Autodesk Inventor part; units mm, degrees
(part 3 of 4)
  spline S572 degree 2 poles (48.1472, 10.9048) (48.1472, 10.1779) (47.354, 9.3436) (46.6302, 9.3436) knots 0 0 0 1 2 2 2
  spline S573 degree 2 poles (46.6302, 9.3436) (45.9096, 9.3436) (45.11, 10.1779) (45.11, 10.9048) knots 0 0 0 1 2 2 2
  spline S574 degree 2 poles (45.11, 10.9048) (45.11, 11.6381) (45.9096, 12.4693) (46.6302, 12.4693) knots 0 0 0 1 2 2 2
  spline S575 degree 2 poles (46.6302, 12.4693) (47.3508, 12.4693) (48.1472, 11.6349) (48.1472, 10.9048) knots 0 0 0 1 2 2 2
  spline S576 degree 2 poles (47.2086, 10.8985) (47.2086, 11.1608) (47.1233, 11.5116) (47.0474, 11.6159) knots 0 0 0 1 2 2 2
  spline S577 degree 2 poles (47.0474, 11.6159) (46.9652, 11.7265) (46.7598, 11.8119) (46.6302, 11.8119) knots 0 0 0 1 2 2 2
  spline S578 degree 2 poles (46.6302, 11.8119) (46.5038, 11.8119) (46.3047, 11.736) (46.2225, 11.6286) knots 0 0 0 1 2 2 2
  spline S579 degree 2 poles (46.2225, 11.6286) (46.1435, 11.5274) (46.0487, 11.1703) (46.0487, 10.8985) knots 0 0 0 1 2 2 2
  spline S580 degree 2 poles (46.0487, 10.8985) (46.0487, 10.6299) (46.1372, 10.298) (46.2099, 10.1969) knots 0 0 0 1 2 2 2
  spline S581 degree 2 poles (46.2099, 10.1969) (46.2826, 10.0958) (46.5038, 10.0009) (46.6365, 10.0009) knots 0 0 0 1 2 2 2
  spline S582 degree 2 poles (46.6365, 10.0009) (46.7472, 10.0009) (46.9747, 10.0958) (47.0442, 10.1906) knots 0 0 0 1 2 2 2
  spline S583 degree 2 poles (47.0442, 10.1906) (47.1233, 10.3012) (47.2086, 10.6204) (47.2086, 10.8985) knots 0 0 0 1 2 2 2
  spline S584 degree 2 poles (53.3746, 10.6299) (53.3746, 10.3391) (53.1534, 9.8998) (52.9701, 9.7544) knots 0 0 0 1 2 2 2
  spline S585 degree 2 poles (52.9701, 9.7544) (52.7489, 9.5806) (52.2242, 9.4352) (51.8165, 9.4352) knots 0 0 0 1 2 2 2
  line L517 (51.8165, 9.4352) -> (50.2584, 9.4352)
  line L518 (50.2584, 9.4352) -> (50.2584, 13.3352)
  line L519 (50.2584, 13.3352) -> (51.6332, 13.3352)
  spline S586 degree 2 poles (51.6332, 13.3352) (52.063, 13.3352) (52.5055, 13.2689) (52.6983, 13.1646) knots 0 0 0 1 2 2 2
  spline S587 degree 2 poles (52.6983, 13.1646) (52.91, 13.0539) (53.1155, 12.6747) (53.1155, 12.4282) knots 0 0 0 1 2 2 2
  spline S588 degree 2 poles (53.1155, 12.4282) (53.1155, 12.1437) (52.831, 11.6981) (52.5782, 11.5938) knots 0 0 0 1 2 2 2
  line L520 (52.5782, 11.5938) -> (52.5782, 11.5748)
  spline S589 degree 2 poles (52.5782, 11.5748) (52.9417, 11.499) (53.3746, 11.0281) (53.3746, 10.6299) knots 0 0 0 1 2 2 2
  spline S590 degree 2 poles (52.3633, 10.6457) (52.3633, 10.829) (52.2179, 11.0344) (52.0725, 11.0881) knots 0 0 0 1 2 2 2
  spline S591 degree 2 poles (52.0725, 11.0881) (51.984, 11.1229) (51.6711, 11.1292) (51.412, 11.1292) knots 0 0 0 1 2 2 2
  line L521 (51.412, 11.1292) -> (51.2318, 11.1292)
  line L522 (51.2318, 11.1292) -> (51.2318, 10.1463)
  line L523 (51.2318, 10.1463) -> (51.2856, 10.1463)
  spline S592 degree 2 poles (51.2856, 10.1463) (51.6648, 10.1463) (51.9556, 10.1558) (52.1073, 10.2222) knots 0 0 0 1 2 2 2
  spline S593 degree 2 poles (52.1073, 10.2222) (52.24, 10.2822) (52.3633, 10.5035) (52.3633, 10.6457) knots 0 0 0 1 2 2 2
  spline S594 degree 2 poles (52.1199, 12.2354) (52.1199, 12.3302) (52.022, 12.5293) (51.9208, 12.5736) knots 0 0 0 1 2 2 2
  spline S595 degree 2 poles (51.9208, 12.5736) (51.826, 12.6178) (51.5605, 12.6241) (51.2982, 12.6241) knots 0 0 0 1 2 2 2
  line L524 (51.2982, 12.6241) -> (51.2318, 12.6241)
  line L525 (51.2318, 12.6241) -> (51.2318, 11.7961)
  line L526 (51.2318, 11.7961) -> (51.3551, 11.7961)
  spline S596 degree 2 poles (51.3551, 11.7961) (51.6048, 11.7961) (51.807, 11.8056) (51.9145, 11.8561) knots 0 0 0 1 2 2 2
  spline S597 degree 2 poles (51.9145, 11.8561) (52.0314, 11.913) (52.1199, 12.1058) (52.1199, 12.2354) knots 0 0 0 1 2 2 2
  spline S598 degree 2 poles (55.391, 9.3562) (54.5566, 9.3562) (53.6686, 10.1526) (53.6686, 10.889) knots 0 0 0 1 2 2 2
  spline S599 degree 2 poles (53.6686, 10.889) (53.6686, 11.6096) (54.4966, 12.4693) (55.2425, 12.4693) knots 0 0 0 1 2 2 2
  spline S600 degree 2 poles (55.2425, 12.4693) (55.9156, 12.4693) (56.5983, 11.7392) (56.5983, 11.0629) knots 0 0 0 1 2 2 2
  line L527 (56.5983, 11.0629) -> (56.5983, 10.731)
  line L528 (56.5983, 10.731) -> (54.5851, 10.731)
  spline S601 degree 2 poles (54.5851, 10.731) (54.5977, 10.5256) (54.7463, 10.2538) (54.8664, 10.1716) knots 0 0 0 1 2 2 2
  spline S602 degree 2 poles (54.8664, 10.1716) (54.9833, 10.0894) (55.2994, 10.0199) (55.4858, 10.0199) knots 0 0 0 1 2 2 2
  spline S603 degree 2 poles (55.4858, 10.0199) (55.6438, 10.0199) (55.9536, 10.0894) (56.0831, 10.1495) knots 0 0 0 1 2 2 2
  spline S604 degree 2 poles (56.0831, 10.1495) (56.1969, 10.1969) (56.3865, 10.3138) (56.4466, 10.3581) knots 0 0 0 1 2 2 2
  line L529 (56.4466, 10.3581) -> (56.5446, 10.3581)
  line L530 (56.5446, 10.3581) -> (56.5446, 9.5996)
  spline S605 degree 2 poles (56.5446, 9.5996) (56.4308, 9.5553) (56.2475, 9.4795) (56.0831, 9.4415) knots 0 0 0 1 2 2 2
  spline S606 degree 2 poles (56.0831, 9.4415) (55.9346, 9.4005) (55.6186, 9.3562) (55.391, 9.3562) knots 0 0 0 1 2 2 2
  spline S607 degree 2 poles (55.6944, 11.2841) (55.6881, 11.5748) (55.4321, 11.8814) (55.1698, 11.8814) knots 0 0 0 1 2 2 2
  spline S608 degree 2 poles (55.1698, 11.8814) (54.9011, 11.8814) (54.5977, 11.559) (54.5819, 11.2841) knots 0 0 0 1 2 2 2
  line L531 (54.5819, 11.2841) -> (55.6944, 11.2841)
  line L532 (59.822, 9.4352) -> (58.8991, 9.4352)
  line L533 (58.8991, 9.4352) -> (58.8991, 10.8922)
  spline S609 degree 2 poles (58.8991, 10.8922) (58.8991, 11.0723) (58.8707, 11.4263) (58.8327, 11.5085) knots 0 0 0 1 2 2 2
  spline S610 degree 2 poles (58.8327, 11.5085) (58.7853, 11.6096) (58.6083, 11.6949) (58.4566, 11.6949) knots 0 0 0 1 2 2 2
  spline S611 degree 2 poles (58.4566, 11.6949) (58.346, 11.6949) (58.1153, 11.6096) (57.9857, 11.518) knots 0 0 0 1 2 2 2
  line L534 (57.9857, 11.518) -> (57.9857, 9.4352)
  line L535 (57.9857, 9.4352) -> (57.0692, 9.4352)
  line L536 (57.0692, 9.4352) -> (57.0692, 12.3776)
  line L537 (57.0692, 12.3776) -> (57.9857, 12.3776)
  line L538 (57.9857, 12.3776) -> (57.9857, 12.0521)
  spline S612 degree 2 poles (57.9857, 12.0521) (58.2101, 12.2417) (58.6368, 12.4566) (58.8959, 12.4566) knots 0 0 0 1 2 2 2
  spline S613 degree 2 poles (58.8959, 12.4566) (59.3447, 12.4566) (59.822, 11.8877) (59.822, 11.3505) knots 0 0 0 1 2 2 2
  line L539 (59.822, 11.3505) -> (59.822, 9.4352)
  spline S614 degree 2 poles (62.009, 9.3562) (61.1746, 9.3562) (60.2865, 10.1526) (60.2865, 10.889) knots 0 0 0 1 2 2 2
  spline S615 degree 2 poles (60.2865, 10.889) (60.2865, 11.6096) (61.1146, 12.4693) (61.8605, 12.4693) knots 0 0 0 1 2 2 2
  spline S616 degree 2 poles (61.8605, 12.4693) (62.5336, 12.4693) (63.2163, 11.7392) (63.2163, 11.0629) knots 0 0 0 1 2 2 2
  line L540 (63.2163, 11.0629) -> (63.2163, 10.731)
  line L541 (63.2163, 10.731) -> (61.2031, 10.731)
  spline S617 degree 2 poles (61.2031, 10.731) (61.2157, 10.5256) (61.3643, 10.2538) (61.4844, 10.1716) knots 0 0 0 1 2 2 2
  spline S618 degree 2 poles (61.4844, 10.1716) (61.6013, 10.0894) (61.9173, 10.0199) (62.1038, 10.0199) knots 0 0 0 1 2 2 2
  spline S619 degree 2 poles (62.1038, 10.0199) (62.2618, 10.0199) (62.5716, 10.0894) (62.7011, 10.1495) knots 0 0 0 1 2 2 2
  spline S620 degree 2 poles (62.7011, 10.1495) (62.8149, 10.1969) (63.0045, 10.3138) (63.0646, 10.3581) knots 0 0 0 1 2 2 2
  line L542 (63.0646, 10.3581) -> (63.1626, 10.3581)
  line L543 (63.1626, 10.3581) -> (63.1626, 9.5996)
  spline S621 degree 2 poles (63.1626, 9.5996) (63.0488, 9.5553) (62.8655, 9.4795) (62.7011, 9.4415) knots 0 0 0 1 2 2 2
  spline S622 degree 2 poles (62.7011, 9.4415) (62.5526, 9.4005) (62.2365, 9.3562) (62.009, 9.3562) knots 0 0 0 1 2 2 2
  spline S623 degree 2 poles (62.3124, 11.2841) (62.3061, 11.5748) (62.0501, 11.8814) (61.7878, 11.8814) knots 0 0 0 1 2 2 2
  spline S624 degree 2 poles (61.7878, 11.8814) (61.5191, 11.8814) (61.2157, 11.559) (61.1999, 11.2841) knots 0 0 0 1 2 2 2
  line L544 (61.1999, 11.2841) -> (62.3124, 11.2841)
  line L545 (66.3609, 9.4352) -> (65.4444, 9.4352)
  line L546 (65.4444, 9.4352) -> (65.4444, 9.7418)
  spline S625 degree 2 poles (65.4444, 9.7418) (65.3559, 9.6691) (65.1284, 9.5016) (65.0399, 9.4573) knots 0 0 0 1 2 2 2
  spline S626 degree 2 poles (65.0399, 9.4573) (64.9324, 9.4068) (64.7175, 9.353) (64.569, 9.353) knots 0 0 0 1 2 2 2
  spline S627 degree 2 poles (64.569, 9.353) (64.0664, 9.353) (63.4786, 10.1874) (63.4786, 10.8827) knots 0 0 0 1 2 2 2
  spline S628 degree 2 poles (63.4786, 10.8827) (63.4786, 11.2683) (63.6777, 11.834) (63.8515, 12.0426) knots 0 0 0 1 2 2 2
  spline S629 degree 2 poles (63.8515, 12.0426) (64.0127, 12.2354) (64.4678, 12.4566) (64.7207, 12.4566) knots 0 0 0 1 2 2 2
  spline S630 degree 2 poles (64.7207, 12.4566) (64.9514, 12.4566) (65.2485, 12.3586) (65.4444, 12.2575) knots 0 0 0 1 2 2 2
  line L547 (65.4444, 12.2575) -> (65.4444, 13.509)
  line L548 (65.4444, 13.509) -> (66.3609, 13.509)
  line L549 (66.3609, 13.509) -> (66.3609, 9.4352)
  line L550 (65.4444, 10.2443) -> (65.4444, 11.6886)
  spline S631 degree 2 poles (65.4444, 11.6886) (65.378, 11.7234) (65.1568, 11.7676) (65.0778, 11.7676) knots 0 0 0 1 2 2 2
  spline S632 degree 2 poles (65.0778, 11.7676) (64.7491, 11.7676) (64.4173, 11.3062) (64.4173, 10.8922) knots 0 0 0 1 2 2 2
  spline S633 degree 2 poles (64.4173, 10.8922) (64.4173, 10.456) (64.6827, 10.0673) (64.9767, 10.0673) knots 0 0 0 1 2 2 2
  spline S634 degree 2 poles (64.9767, 10.0673) (65.0968, 10.0673) (65.3433, 10.1621) (65.4444, 10.2443) knots 0 0 0 1 2 2 2
  line L551 (69.7932, 9.4352) -> (68.8767, 9.4352)
  line L552 (68.8767, 9.4352) -> (68.8767, 9.7607)
  spline S635 degree 2 poles (68.8767, 9.7607) (68.6396, 9.5616) (68.2414, 9.353) (67.9664, 9.353) knots 0 0 0 1 2 2 2
  spline S636 degree 2 poles (67.9664, 9.353) (67.5303, 9.353) (67.0404, 9.9061) (67.0404, 10.4624) knots 0 0 0 1 2 2 2
  line L553 (67.0404, 10.4624) -> (67.0404, 12.3776)
  line L554 (67.0404, 12.3776) -> (67.9633, 12.3776)
  line L555 (67.9633, 12.3776) -> (67.9633, 10.9175)
  spline S637 degree 2 poles (67.9633, 10.9175) (67.9633, 10.6899) (67.9854, 10.3992) (68.0297, 10.3012) knots 0 0 0 1 2 2 2
  spline S638 degree 2 poles (68.0297, 10.3012) (68.0739, 10.2095) (68.2477, 10.1147) (68.4058, 10.1147) knots 0 0 0 1 2 2 2
  spline S639 degree 2 poles (68.4058, 10.1147) (68.5006, 10.1147) (68.766, 10.2095) (68.8767, 10.2917) knots 0 0 0 1 2 2 2
  line L556 (68.8767, 10.2917) -> (68.8767, 12.3776)
  line L557 (68.8767, 12.3776) -> (69.7932, 12.3776)
  line L558 (69.7932, 12.3776) -> (69.7932, 9.4352)
  spline S640 degree 2 poles (71.936, 9.3562) (71.5725, 9.3562) (70.9689, 9.5395) (70.7445, 9.7291) knots 0 0 0 1 2 2 2
  spline S641 degree 2 poles (70.7445, 9.7291) (70.5264, 9.9219) (70.2799, 10.5003) (70.2799, 10.8922) knots 0 0 0 1 2 2 2
  spline S642 degree 2 poles (70.2799, 10.8922) (70.2799, 11.3157) (70.5454, 11.9067) (70.7761, 12.0963) knots 0 0 0 1 2 2 2
  spline S643 degree 2 poles (70.7761, 12.0963) (70.9942, 12.2796) (71.5883, 12.4566) (71.9107, 12.4566) knots 0 0 0 1 2 2 2
  spline S644 degree 2 poles (71.9107, 12.4566) (72.1541, 12.4566) (72.6408, 12.3428) (72.8873, 12.2196) knots 0 0 0 1 2 2 2
  line L559 (72.8873, 12.2196) -> (72.8873, 11.4358)
  line L560 (72.8873, 11.4358) -> (72.7703, 11.4358)
  spline S645 degree 2 poles (72.7703, 11.4358) (72.7135, 11.4895) (72.5554, 11.6159) (72.4606, 11.6665) knots 0 0 0 1 2 2 2
  spline S646 degree 2 poles (72.4606, 11.6665) (72.3595, 11.7234) (72.1098, 11.7992) (71.9549, 11.7992) knots 0 0 0 1 2 2 2
  spline S647 degree 2 poles (71.9549, 11.7992) (71.6041, 11.7992) (71.2186, 11.3094) (71.2186, 10.8922) knots 0 0 0 1 2 2 2
  spline S648 degree 2 poles (71.2186, 10.8922) (71.2186, 10.4497) (71.6294, 10.0136) (71.9707, 10.0136) knots 0 0 0 1 2 2 2
  spline S649 degree 2 poles (71.9707, 10.0136) (72.1446, 10.0136) (72.4037, 10.0926) (72.4985, 10.1495) knots 0 0 0 1 2 2 2
  spline S650 degree 2 poles (72.4985, 10.1495) (72.5902, 10.2032) (72.7229, 10.3233) (72.7703, 10.3707) knots 0 0 0 1 2 2 2
  line L561 (72.7703, 10.3707) -> (72.8873, 10.3707)
  line L562 (72.8873, 10.3707) -> (72.8873, 9.5838)
  spline S651 degree 2 poles (72.8873, 9.5838) (72.8083, 9.549) (72.6028, 9.4605) (72.4954, 9.4321) knots 0 0 0 1 2 2 2
  spline S652 degree 2 poles (72.4954, 9.4321) (72.3626, 9.3941) (72.1288, 9.3562) (71.936, 9.3562) knots 0 0 0 1 2 2 2
  spline S653 degree 2 poles (74.831, 9.3562) (73.9966, 9.3562) (73.1085, 10.1526) (73.1085, 10.889) knots 0 0 0 1 2 2 2
  spline S654 degree 2 poles (73.1085, 10.889) (73.1085, 11.6096) (73.9365, 12.4693) (74.6824, 12.4693) knots 0 0 0 1 2 2 2
  spline S655 degree 2 poles (74.6824, 12.4693) (75.3556, 12.4693) (76.0382, 11.7392) (76.0382, 11.0629) knots 0 0 0 1 2 2 2
  line L563 (76.0382, 11.0629) -> (76.0382, 10.731)
  line L564 (76.0382, 10.731) -> (74.025, 10.731)
  spline S656 degree 2 poles (74.025, 10.731) (74.0377, 10.5256) (74.1862, 10.2538) (74.3063, 10.1716) knots 0 0 0 1 2 2 2
  spline S657 degree 2 poles (74.3063, 10.1716) (74.4233, 10.0894) (74.7393, 10.0199) (74.9258, 10.0199) knots 0 0 0 1 2 2 2
  spline S658 degree 2 poles (74.9258, 10.0199) (75.0838, 10.0199) (75.3935, 10.0894) (75.5231, 10.1495) knots 0 0 0 1 2 2 2
  spline S659 degree 2 poles (75.5231, 10.1495) (75.6369, 10.1969) (75.8265, 10.3138) (75.8865, 10.3581) knots 0 0 0 1 2 2 2
  line L565 (75.8865, 10.3581) -> (75.9845, 10.3581)
  line L566 (75.9845, 10.3581) -> (75.9845, 9.5996)
  spline S660 degree 2 poles (75.9845, 9.5996) (75.8707, 9.5553) (75.6874, 9.4795) (75.5231, 9.4415) knots 0 0 0 1 2 2 2
  spline S661 degree 2 poles (75.5231, 9.4415) (75.3746, 9.4005) (75.0585, 9.3562) (74.831, 9.3562) knots 0 0 0 1 2 2 2
  spline S662 degree 2 poles (75.1344, 11.2841) (75.128, 11.5748) (74.872, 11.8814) (74.6097, 11.8814) knots 0 0 0 1 2 2 2
  spline S663 degree 2 poles (74.6097, 11.8814) (74.3411, 11.8814) (74.0377, 11.559) (74.0219, 11.2841) knots 0 0 0 1 2 2 2
  line L567 (74.0219, 11.2841) -> (75.1344, 11.2841)
  line L568 (81.4742, 9.4352) -> (80.5324, 9.4352)
  line L569 (80.5324, 9.4352) -> (79.028, 12.1532)
  line L570 (79.028, 12.1532) -> (79.028, 9.4352)
  line L571 (79.028, 9.4352) -> (78.1336, 9.4352)
  line L572 (78.1336, 9.4352) -> (78.1336, 13.3352)
  line L573 (78.1336, 13.3352) -> (79.3346, 13.3352)
  line L574 (79.3346, 13.3352) -> (80.5798, 11.1008)
  line L575 (80.5798, 11.1008) -> (80.5798, 13.3352)
  line L576 (80.5798, 13.3352) -> (81.4742, 13.3352)
  line L577 (81.4742, 13.3352) -> (81.4742, 9.4352)
  spline S664 degree 2 poles (83.7213, 9.3562) (82.887, 9.3562) (81.9989, 10.1526) (81.9989, 10.889) knots 0 0 0 1 2 2 2
  spline S665 degree 2 poles (81.9989, 10.889) (81.9989, 11.6096) (82.8269, 12.4693) (83.5728, 12.4693) knots 0 0 0 1 2 2 2
  spline S666 degree 2 poles (83.5728, 12.4693) (84.2459, 12.4693) (84.9286, 11.7392) (84.9286, 11.0629) knots 0 0 0 1 2 2 2
  line L578 (84.9286, 11.0629) -> (84.9286, 10.731)
  line L579 (84.9286, 10.731) -> (82.9154, 10.731)
  spline S667 degree 2 poles (82.9154, 10.731) (82.928, 10.5256) (83.0766, 10.2538) (83.1967, 10.1716) knots 0 0 0 1 2 2 2
  spline S668 degree 2 poles (83.1967, 10.1716) (83.3136, 10.0894) (83.6297, 10.0199) (83.8161, 10.0199) knots 0 0 0 1 2 2 2
  spline S669 degree 2 poles (83.8161, 10.0199) (83.9741, 10.0199) (84.2839, 10.0894) (84.4135, 10.1495) knots 0 0 0 1 2 2 2
  spline S670 degree 2 poles (84.4135, 10.1495) (84.5272, 10.1969) (84.7169, 10.3138) (84.7769, 10.3581) knots 0 0 0 1 2 2 2
  line L580 (84.7769, 10.3581) -> (84.8749, 10.3581)
  line L581 (84.8749, 10.3581) -> (84.8749, 9.5996)
  spline S671 degree 2 poles (84.8749, 9.5996) (84.7611, 9.5553) (84.5778, 9.4795) (84.4135, 9.4415) knots 0 0 0 1 2 2 2
  spline S672 degree 2 poles (84.4135, 9.4415) (84.2649, 9.4005) (83.9489, 9.3562) (83.7213, 9.3562) knots 0 0 0 1 2 2 2
  spline S673 degree 2 poles (84.0247, 11.2841) (84.0184, 11.5748) (83.7624, 11.8814) (83.5001, 11.8814) knots 0 0 0 1 2 2 2
  spline S674 degree 2 poles (83.5001, 11.8814) (83.2314, 11.8814) (82.928, 11.559) (82.9122, 11.2841) knots 0 0 0 1 2 2 2
  line L582 (82.9122, 11.2841) -> (84.0247, 11.2841)
  spline S675 degree 2 poles (86.5246, 9.3783) (85.9652, 9.3783) (85.4532, 9.8398) (85.4532, 10.3644) knots 0 0 0 1 2 2 2
  line L583 (85.4532, 10.3644) -> (85.4532, 11.7392)
  line L584 (85.4532, 11.7392) -> (85.1024, 11.7392)
  line L585 (85.1024, 11.7392) -> (85.1024, 12.3776)
  line L586 (85.1024, 12.3776) -> (85.4532, 12.3776)
  line L587 (85.4532, 12.3776) -> (85.4532, 13.2183)
  line L588 (85.4532, 13.2183) -> (86.3698, 13.2183)
  line L589 (86.3698, 13.2183) -> (86.3698, 12.3776)
  line L590 (86.3698, 12.3776) -> (87.2547, 12.3776)
  line L591 (87.2547, 12.3776) -> (87.2547, 11.7392)
  line L592 (87.2547, 11.7392) -> (86.3698, 11.7392)
  line L593 (86.3698, 11.7392) -> (86.3698, 10.6931)
  spline S676 degree 2 poles (86.3698, 10.6931) (86.3698, 10.5382) (86.3761, 10.3075) (86.414, 10.2159) knots 0 0 0 1 2 2 2
  spline S677 degree 2 poles (86.414, 10.2159) (86.4519, 10.1242) (86.6384, 10.0167) (86.8154, 10.0167) knots 0 0 0 1 2 2 2
  spline S678 degree 2 poles (86.8154, 10.0167) (86.8912, 10.0167) (87.1283, 10.08) (87.1757, 10.1052) knots 0 0 0 1 2 2 2
  line L594 (87.1757, 10.1052) -> (87.2547, 10.1052)
  line L595 (87.2547, 10.1052) -> (87.2547, 9.4605)
  spline S679 degree 2 poles (87.2547, 9.4605) (87.1062, 9.4226) (86.7711, 9.3783) (86.5246, 9.3783) knots 0 0 0 1 2 2 2
  spline S680 degree 2 poles (90.4499, 10.9048) (90.4499, 10.1779) (89.6566, 9.3436) (88.9329, 9.3436) knots 0 0 0 1 2 2 2
  spline S681 degree 2 poles (88.9329, 9.3436) (88.2123, 9.3436) (87.4127, 10.1779) (87.4127, 10.9048) knots 0 0 0 1 2 2 2
  spline S682 degree 2 poles (87.4127, 10.9048) (87.4127, 11.6381) (88.2123, 12.4693) (88.9329, 12.4693) knots 0 0 0 1 2 2 2
  spline S683 degree 2 poles (88.9329, 12.4693) (89.6535, 12.4693) (90.4499, 11.6349) (90.4499, 10.9048) knots 0 0 0 1 2 2 2
  spline S684 degree 2 poles (89.5113, 10.8985) (89.5113, 11.1608) (89.4259, 11.5116) (89.3501, 11.6159) knots 0 0 0 1 2 2 2
  spline S685 degree 2 poles (89.3501, 11.6159) (89.2679, 11.7265) (89.0625, 11.8119) (88.9329, 11.8119) knots 0 0 0 1 2 2 2
  spline S686 degree 2 poles (88.9329, 11.8119) (88.8065, 11.8119) (88.6074, 11.736) (88.5252, 11.6286) knots 0 0 0 1 2 2 2
  spline S687 degree 2 poles (88.5252, 11.6286) (88.4462, 11.5274) (88.3514, 11.1703) (88.3514, 10.8985) knots 0 0 0 1 2 2 2
  spline S688 degree 2 poles (88.3514, 10.8985) (88.3514, 10.6299) (88.4399, 10.298) (88.5126, 10.1969) knots 0 0 0 1 2 2 2
  spline S689 degree 2 poles (88.5126, 10.1969) (88.5852, 10.0958) (88.8065, 10.0009) (88.9392, 10.0009) knots 0 0 0 1 2 2 2
  spline S690 degree 2 poles (88.9392, 10.0009) (89.0498, 10.0009) (89.2774, 10.0958) (89.3469, 10.1906) knots 0 0 0 1 2 2 2
  spline S691 degree 2 poles (89.3469, 10.1906) (89.4259, 10.3012) (89.5113, 10.6204) (89.5113, 10.8985) knots 0 0 0 1 2 2 2
  line L596 (44.4187, 2.6614) -> (41.5521, 2.6614)
  line L597 (41.5521, 2.6614) -> (41.5521, 3.2967)
  spline S692 degree 2 poles (41.5521, 3.2967) (41.9156, 3.5874) (42.4971, 4.0994) (42.7152, 4.3302) knots 0 0 0 1 2 2 2
  spline S693 degree 2 poles (42.7152, 4.3302) (43.0028, 4.6304) (43.2588, 5.0887) (43.2588, 5.3289) knots 0 0 0 1 2 2 2
  spline S694 degree 2 poles (43.2588, 5.3289) (43.2588, 5.6007) (42.9333, 5.8914) (42.6425, 5.8914) knots 0 0 0 1 2 2 2
  spline S695 degree 2 poles (42.6425, 5.8914) (42.4939, 5.8914) (42.2285, 5.8187) (42.0926, 5.7618) knots 0 0 0 1 2 2 2
  spline S696 degree 2 poles (42.0926, 5.7618) (41.9598, 5.7018) (41.7702, 5.5754) (41.7228, 5.5438) knots 0 0 0 1 2 2 2
  line L598 (41.7228, 5.5438) -> (41.6469, 5.5438)
  line L599 (41.6469, 5.5438) -> (41.6469, 6.3939)
  spline S697 degree 2 poles (41.6469, 6.3939) (41.8113, 6.4729) (42.5129, 6.6373) (42.8384, 6.6373) knots 0 0 0 1 2 2 2
  spline S698 degree 2 poles (42.8384, 6.6373) (43.5337, 6.6373) (44.248, 6.0178) (44.248, 5.4584) knots 0 0 0 1 2 2 2
  spline S699 degree 2 poles (44.248, 5.4584) (44.248, 5.1139) (43.9225, 4.4502) (43.5464, 4.071) knots 0 0 0 1 2 2 2
  spline S700 degree 2 poles (43.5464, 4.071) (43.3093, 3.8371) (42.8637, 3.4737) (42.7657, 3.3978) knots 0 0 0 1 2 2 2
  line L600 (42.7657, 3.3978) -> (44.4187, 3.3978)
  line L601 (44.4187, 3.3978) -> (44.4187, 2.6614)
  spline S701 degree 2 poles (47.7845, 4.6114) (47.7845, 4.1058) (47.6234, 3.3473) (47.4432, 3.0913) knots 0 0 0 1 2 2 2
  spline S702 degree 2 poles (47.4432, 3.0913) (47.2662, 2.8384) (46.6942, 2.5793) (46.2833, 2.5793) knots 0 0 0 1 2 2 2
  spline S703 degree 2 poles (46.2833, 2.5793) (45.8693, 2.5793) (45.3004, 2.8384) (45.1203, 3.0976) knots 0 0 0 1 2 2 2
  spline S704 degree 2 poles (45.1203, 3.0976) (44.9401, 3.3536) (44.779, 4.1058) (44.779, 4.6114) knots 0 0 0 1 2 2 2
  spline S705 degree 2 poles (44.779, 4.6114) (44.779, 5.1297) (44.9401, 5.863) (45.1234, 6.1284) knots 0 0 0 1 2 2 2
  spline S706 degree 2 poles (45.1234, 6.1284) (45.3068, 6.3876) (45.8851, 6.6404) (46.2833, 6.6404) knots 0 0 0 1 2 2 2
  spline S707 degree 2 poles (46.2833, 6.6404) (46.7037, 6.6404) (47.2662, 6.375) (47.4464, 6.1126) knots 0 0 0 1 2 2 2
  spline S708 degree 2 poles (47.4464, 6.1126) (47.6234, 5.8567) (47.7845, 5.1013) (47.7845, 4.6114) knots 0 0 0 1 2 2 2
  spline S709 degree 2 poles (46.8016, 4.6114) (46.8016, 5.3352) (46.5646, 5.9199) (46.2833, 5.9199) knots 0 0 0 1 2 2 2
  spline S710 degree 2 poles (46.2833, 5.9199) (46.0021, 5.9199) (45.7619, 5.3352) (45.7619, 4.6083) knots 0 0 0 1 2 2 2
  spline S711 degree 2 poles (45.7619, 4.6083) (45.7619, 3.894) (46.0021, 3.2998) (46.2833, 3.2998) knots 0 0 0 1 2 2 2
  spline S712 degree 2 poles (46.2833, 3.2998) (46.5615, 3.2998) (46.8016, 3.894) (46.8016, 4.6114) knots 0 0 0 1 2 2 2
  line L602 (51.2516, 2.6614) -> (48.385, 2.6614)
  line L603 (48.385, 2.6614) -> (48.385, 3.2967)
  spline S713 degree 2 poles (48.385, 3.2967) (48.7485, 3.5874) (49.33, 4.0994) (49.5481, 4.3302) knots 0 0 0 1 2 2 2
  spline S714 degree 2 poles (49.5481, 4.3302) (49.8357, 4.6304) (50.0917, 5.0887) (50.0917, 5.3289) knots 0 0 0 1 2 2 2
  spline S715 degree 2 poles (50.0917, 5.3289) (50.0917, 5.6007) (49.7662, 5.8914) (49.4754, 5.8914) knots 0 0 0 1 2 2 2
  spline S716 degree 2 poles (49.4754, 5.8914) (49.3268, 5.8914) (49.0614, 5.8187) (48.9255, 5.7618) knots 0 0 0 1 2 2 2
  spline S717 degree 2 poles (48.9255, 5.7618) (48.7927, 5.7018) (48.6031, 5.5754) (48.5557, 5.5438) knots 0 0 0 1 2 2 2
  line L604 (48.5557, 5.5438) -> (48.4798, 5.5438)
  line L605 (48.4798, 5.5438) -> (48.4798, 6.3939)
  spline S718 degree 2 poles (48.4798, 6.3939) (48.6442, 6.4729) (49.3458, 6.6373) (49.6713, 6.6373) knots 0 0 0 1 2 2 2
  spline S719 degree 2 poles (49.6713, 6.6373) (50.3666, 6.6373) (51.0809, 6.0178) (51.0809, 5.4584) knots 0 0 0 1 2 2 2
  spline S720 degree 2 poles (51.0809, 5.4584) (51.0809, 5.1139) (50.7554, 4.4502) (50.3793, 4.071) knots 0 0 0 1 2 2 2
  spline S721 degree 2 poles (50.3793, 4.071) (50.1422, 3.8371) (49.6966, 3.4737) (49.5986, 3.3978) knots 0 0 0 1 2 2 2
  line L606 (49.5986, 3.3978) -> (51.2516, 3.3978)
  line L607 (51.2516, 3.3978) -> (51.2516, 2.6614)
  line L608 (54.668, 2.6614) -> (51.8015, 2.6614)
  line L609 (51.8015, 2.6614) -> (51.8015, 3.2967)
  spline S722 degree 2 poles (51.8015, 3.2967) (52.1649, 3.5874) (52.7465, 4.0994) (52.9645, 4.3302) knots 0 0 0 1 2 2 2
  spline S723 degree 2 poles (52.9645, 4.3302) (53.2521, 4.6304) (53.5081, 5.0887) (53.5081, 5.3289) knots 0 0 0 1 2 2 2
  spline S724 degree 2 poles (53.5081, 5.3289) (53.5081, 5.6007) (53.1826, 5.8914) (52.8918, 5.8914) knots 0 0 0 1 2 2 2
  spline S725 degree 2 poles (52.8918, 5.8914) (52.7433, 5.8914) (52.4778, 5.8187) (52.3419, 5.7618) knots 0 0 0 1 2 2 2
  spline S726 degree 2 poles (52.3419, 5.7618) (52.2092, 5.7018) (52.0196, 5.5754) (51.9721, 5.5438) knots 0 0 0 1 2 2 2
  line L610 (51.9721, 5.5438) -> (51.8963, 5.5438)
  line L611 (51.8963, 5.5438) -> (51.8963, 6.3939)
  spline S727 degree 2 poles (51.8963, 6.3939) (52.0606, 6.4729) (52.7623, 6.6373) (53.0878, 6.6373) knots 0 0 0 1 2 2 2
  spline S728 degree 2 poles (53.0878, 6.6373) (53.7831, 6.6373) (54.4974, 6.0178) (54.4974, 5.4584) knots 0 0 0 1 2 2 2
  spline S729 degree 2 poles (54.4974, 5.4584) (54.4974, 5.1139) (54.1718, 4.4502) (53.7957, 4.071) knots 0 0 0 1 2 2 2
  spline S730 degree 2 poles (53.7957, 4.071) (53.5587, 3.8371) (53.1131, 3.4737) (53.0151, 3.3978) knots 0 0 0 1 2 2 2
  line L612 (53.0151, 3.3978) -> (54.668, 3.3978)
  line L613 (54.668, 3.3978) -> (54.668, 2.6614)
  point P0 (0, 0)
  constraints: 10 other
extrude "Extrusão3" cut sketch "Esboço2" against normal blind 0.8
chamfer "Chanfro1" distance 4 angle 45 4 edges at (1, 40, -100) (1, 0, -100) (1, 40, 0) (1, 0, 0)
fillet "Arredondamento1" radius 2 8 edges at (1, 40, -4) (1, 36, 0) (1, 4, 0) (1, 0, -4) (1, 0, -96) (1, 4, -100) (1, 36, -100) (1, 40, -96)
sketch "Esboço4" plane through (2, 0, 0) normal (1, 0, 0) x (0, 0, -1)
  line L0 (45.497, 3.0913) -> (45.497, 2.5793) projected
  line L1 (46.2833, 8.4074) -> (45.1203, 8.4074) projected
  line L2 (45.0667, 6.1126) -> (45.0667, 4.6114) projected
  line L3 (47.7845, 11.4269) -> (47.4432, 11.4269) projected
  line L4 (88.9329, 10.6586) -> (88.5252, 10.6586) projected
  line L5 (50.5558, 25.9389) -> (50.2933, 25.2422) projected
  line L6 (88.3514, 8.4074) -> (88.5126, 8.4074) projected
  line L7 (49.6589, 25.5886) -> (49.6742, 25.6323) projected
  line L8 (40.3066, 9.4415) -> (40.3066, 9.3562) projected
  line L9 (83.7213, 8.4074) -> (81.9989, 8.4074) projected
  line L10 (84.8749, 10.3581) -> (84.8749, 9.5996) projected
  line L11 (40.8378, 9.5996) -> (40.8378, 9.4415) projected
  line L12 (35.8187, 11.2841) -> (35.8187, 11.8814) projected
  line L13 (74.6097, 8.4074) -> (74.0219, 8.4074) projected
  line L14 (74.0219, 11.2841) -> (75.1344, 11.2841) projected
  line L15 (32.3678, 11.7676) -> (32.3678, 10.8922) projected
  line L16 (64.4173, 8.4074) -> (64.9767, 8.4074) projected
  line L17 (65.4444, 10.2443) -> (65.4444, 11.6886) projected
  line L18 (65.4444, 8.9812) -> (65.0778, 8.9812) projected
  line L19 (58.8991, 9.4352) -> (58.8991, 10.8922) projected
  line L20 (58.8991, 10.6708) -> (58.8327, 10.6708) projected
  line L21 (57.9857, 11.518) -> (57.9857, 9.4352) projected
  line L22 (57.9857, 9.4352) -> (57.0692, 9.4352) projected
  line L23 (57.9857, 12.3776) -> (57.9857, 12.0521) projected
  line L24 (25.9107, 12.0521) -> (25.9107, 12.4566) projected
  line L25 (58.8959, 11.0087) -> (59.822, 11.0087) projected
  line L26 (56.5446, 9.5257) -> (56.0831, 9.5257) projected
  line L27 (21.5189, 9.4415) -> (21.5189, 9.3562) projected
  line L28 (55.391, 8.4074) -> (53.6686, 8.4074) projected
  line L29 (66.2594, 10.6457) -> (66.2594, 11.0881) projected
  line L30 (66.6387, 10.1463) -> (66.6387, 10.2222) projected
  line L31 (52.1073, 15.7473) -> (52.3633, 15.7473) projected
  line L32 (64.4482, 11.6286) -> (64.4482, 10.8985) projected
  line L33 (46.0487, 15.7473) -> (46.2099, 15.7473) projected
  line L34 (64.069, 11.6159) -> (64.069, 11.8119) projected
  line L35 (68.4085, 11.8119) -> (68.4085, 11.6286) projected
  line L36 (41.2985, 9.4352) -> (40.2524, 12.3776) projected
  line L37 (40.2524, 12.3776) -> (41.2164, 12.3776) projected
  line L38 (41.2164, 12.3776) -> (41.8169, 10.4339) projected
  line L39 (41.8169, 10.4339) -> (42.411, 12.3776) projected
  line L40 (42.411, 12.3776) -> (43.356, 12.3776) projected
  line L41 (43.356, 12.3776) -> (42.3004, 9.4352) projected
  line L42 (42.3004, 9.4352) -> (41.2985, 9.4352) projected
  line L43 (38.0464, 12.7948) -> (38.59, 13.8251) projected
  line L44 (24.0772, 12.6083) -> (24.0583, 12.6083) projected
  line L45 (24.0583, 12.6083) -> (24.0583, 10.1653) projected
  line L46 (44.6395, 11.3884) -> (44.6395, 12.4787) projected
  line L47 (25.0159, 18.881) -> (24.0772, 18.881) projected
  line L48 (19.8011, 9.4352) -> (19.8011, 10.4655) projected
  line L49 (41.9045, 11.6286) -> (41.9045, 10.8985) projected
  line L50 (15.1426, 15.7473) -> (15.3038, 15.7473) projected
  line L51 (15.7241, 17.167) -> (15.3165, 17.167) projected
  line L52 (72.3511, 18.8786) -> (73.4036, 18.8786) projected
  line L53 (36.6071, 18.9065) -> (36.6071, 17.8825) projected
  line L54 (74.8574, 17.8825) -> (74.8574, 15.882) projected
  line L55 (74.8574, 15.882) -> (73.9472, 15.882) projected
  line L56 (73.9472, 15.882) -> (73.9472, 16.1949) projected
  line L57 (66.3178, 25.1305) -> (66.7919, 25.1305) projected
  line L58 (66.7919, 16.65) -> (66.7919, 17.2599) projected
  line L59 (62.1081, 15.882) -> (62.1081, 19.782) projected
  line L60 (62.1081, 19.782) -> (64.7186, 19.782) projected
  line L61 (63.0815, 18.3029) -> (64.5891, 18.3029) projected
  line L62 (64.5891, 18.3029) -> (64.5891, 17.5602) projected
  line L63 (85.5491, 15.9262) -> (85.5491, 15.803) projected
  line L64 (57.9584, 27.0186) -> (57.0514, 27.0186) projected
  line L65 (58.8939, 25.5562) -> (58.5242, 25.5562) projected
  line L66 (89.428, 18.0279) -> (89.428, 17.7561) projected
  line L67 (53.3979, 26.3683) -> (53.9636, 26.3683) projected
  line L68 (88.8891, 16.0937) -> (88.8891, 15.803) projected
  line L69 (53.1798, 24.371) -> (52.0895, 24.371) projected
  line L70 (54.4788, 18.6948) -> (54.4788, 17.9489) projected
  line L71 (54.4788, 17.9489) -> (54.4061, 17.9489) projected
  line L72 (84.2808, 17.9489) -> (84.2808, 18.1543) projected
  line L73 (41.6821, 16.8048) -> (41.6821, 16.0463) projected
  line L74 (38.3194, 18.8244) -> (38.3194, 15.882) projected
  line L75 (38.3194, 15.882) -> (37.4028, 15.882) projected
  line L76 (37.4028, 15.882) -> (37.4028, 18.8244) projected
  line L77 (37.4028, 18.8244) -> (38.3194, 18.8244) projected
  line L78 (70.8185, 17.8509) -> (70.8185, 16.5172) projected
  line L79 (26.0884, 18.0248) -> (27.7919, 18.0248) projected
  line L80 (70.0426, 26.2811) -> (70.0426, 27.6851) projected
  line L81 (68.6508, 24.88) -> (68.6508, 26.2811) projected
  line L82 (68.8544, 31.0829) -> (68.8334, 30.9922) projected
  line L83 (92.7017, 26.7067) -> (93.0251, 26.7067) projected
  line L84 (93.0251, 25.5636) -> (93.096, 25.5636) projected
  line L85 (66.7505, 24.9112) -> (66.7505, 25.7961) projected
  line L86 (63.5616, 25.6033) -> (63.5616, 25.7905) projected
  line L87 (62.8141, 24.9679) -> (62.8141, 24.8914) projected
  line L88 (89.925, 24.8306) -> (88.3792, 24.8306) projected
  line L89 (81.2658, 26.7293) -> (81.2658, 24.9623) projected
  line L90 (81.2658, 24.9623) -> (80.4432, 24.9623) projected
  line L91 (58.0936, 26.8229) -> (58.0936, 26.8569) projected
  line L92 (81.8132, 25.3088) -> (81.2658, 25.3088) projected
  line L93 (57.9312, 31.4149) -> (57.5522, 29.7853) projected
  line L94 (78.645, 24.8306) -> (77.2808, 24.8306) projected
  line L95 (52.5872, 26.1989) -> (52.5872, 26.1025) projected
  line L96 (53.5284, 26.1025) -> (53.5284, 25.7876) projected
  line L97 (50.6787, 27.6057) -> (50.6787, 26.7066) projected
  line L98 (70.6778, 27.0186) -> (70.9927, 27.0186) projected
  line L99 (72.2009, 24.371) -> (71.6252, 24.371) projected
  line L100 (51.9036, 27.8751) -> (51.9036, 27.6057) projected
  line L101 (62.7532, 26.2572) -> (62.3675, 26.2572) projected
  line L102 (46.6626, 26.3691) -> (46.6626, 26.5421) projected
  line L103 (61.942, 24.371) -> (61.7066, 24.371) projected
  line L104 (46.075, 25.5721) -> (46.075, 25.8982) projected
  line L105 (45.1682, 27.9461) -> (45.1682, 27.6114) projected
  line L106 (43.9741, 27.6114) -> (43.9741, 27.2285) projected
  line L107 (44.7671, 27.0668) -> (44.7671, 27.5546) projected
  line L108 (59.6106, 26.7067) -> (59.1738, 26.7067) projected
  line L109 (54.2925, 25.1305) -> (53.8983, 25.1305) projected
  line L110 (39.7711, 24.2447) -> (39.7711, 23.9696) projected
  line L111 (45.3468, 26.8314) -> (45.3468, 24.9623) projected
  line L112 (45.3468, 24.9623) -> (44.5243, 24.9623) projected
  line L113 (46.0502, 24.8005) -> (45.7325, 24.8005) projected
  line L114 (34.5252, 26.9902) -> (34.5252, 26.8314) projected
  line L115 (30.2951, 26.2811) -> (30.2951, 24.88) projected
  line L116 (42.7289, 24.371) -> (41.3646, 24.371) projected
  line L117 (37.5356, 24.9623) -> (37.5356, 25.8869) projected
  line L118 (23.4108, 25.7933) -> (23.4108, 26.9902) projected
  line L119 (21.0244, 25.8302) -> (21.0244, 25.6486) projected
  line L120 (22.991, 24.371) -> (23.4108, 24.371) projected
  line L121 (21.0879, 28.6183) -> (19.6953, 24.2021) projected
  line L122 (19.6953, 24.2021) -> (19.0202, 24.2021) projected
  line L123 (14.6778, 26.6782) -> (14.6778, 27.6029) projected
  line L124 (10.0033, 26.6442) -> (10.0033, 26.5279) projected
  line L125 (13.5632, 24.371) -> (14.1418, 24.371) projected
  line L126 (9.4158, 25.7876) -> (9.4158, 25.1523) projected
  line L127 (8.2387, 27.4128) -> (8.2387, 27.6738) projected
  line L128 (13.1235, 26.2572) -> (14.0255, 26.2572) projected
  line L129 (14.0255, 27.4866) -> (14.0255, 26.8172) projected
  line L130 (9.4158, 27.1093) -> (9.4158, 26.8881) projected
  line L131 (12.7293, 26.2572) -> (13.0555, 26.2572) projected
  line L132 (70.2629, 35.4864) -> (70.2629, 34.2607) projected
  line L133 (70.2629, 34.2607) -> (70.1559, 34.2607) projected
  line L134 (68.7698, 34.1136) -> (68.7698, 31.3369) projected
  line L135 (68.7698, 31.3369) -> (67.4772, 31.3369) projected
  line L136 (67.4772, 35.4864) -> (68.7698, 35.4864) projected
  line L137 (68.7698, 35.4864) -> (68.7698, 34.8891) projected
  line L138 (62.7924, 34.8891) -> (62.7924, 35.2947) projected
  line L139 (58.884, 34.0378) -> (58.884, 31.3369) projected
  line L140 (58.884, 31.3369) -> (57.5826, 31.3369) projected
  line L141 (56.4059, 34.2741) -> (56.4059, 31.3369) projected
  line L142 (56.4059, 31.3369) -> (55.1044, 31.3369) projected
  line L143 (55.1044, 31.3369) -> (55.1044, 33.4094) projected
  line L144 (53.9189, 34.2741) -> (53.9189, 31.3369) projected
  line L145 (53.9189, 31.3369) -> (52.6263, 31.3369) projected
  line L146 (52.6263, 31.3369) -> (52.6263, 35.4864) projected
  line L147 (52.6263, 35.4864) -> (53.9189, 35.4864) projected
  line L148 (55.3532, 35.2279) -> (55.3532, 34.0378) projected
  line L149 (51.6413, 35.4864) -> (51.6413, 31.3369) projected
  line L150 (51.6413, 31.3369) -> (50.3488, 31.3369) projected
  line L151 (50.3488, 31.3369) -> (50.3488, 35.4864) projected
  line L152 (50.3488, 35.4864) -> (51.6413, 35.4864) projected
  line L153 (41.4124, 37.082) -> (41.4124, 31.3369) projected
  line L154 (41.4124, 31.3369) -> (40.1198, 31.3369) projected
  line L155 (40.1198, 31.3369) -> (40.1198, 37.082) projected
  line L156 (40.1198, 37.082) -> (41.4124, 37.082) projected
  line L157 (37.8779, 31.3369) -> (37.8779, 31.7781) projected
  line L158 (39.5914, 32.5269) -> (39.5914, 33.7214) projected
  line L159 (36.8706, 34.2748) -> (35.7386, 34.2748) projected
  line L160 (35.7386, 34.3944) -> (35.6271, 34.3944) projected
  line L161 (39.1616, 34.1582) -> (39.1616, 31.3369) projected
  line L162 (39.1616, 31.3369) -> (37.8779, 31.3369) projected
  line L163 (34.7268, 32.9949) -> (34.8516, 32.9949) projected
  line L164 (34.8516, 32.9949) -> (34.8516, 31.7023) projected
  line L165 (34.7134, 32.3826) -> (34.1162, 32.3826) projected
  line L166 (36.9294, 35.629) -> (36.9294, 35.9143) projected
  line L167 (49.854, 35.4864) -> (49.854, 34.2607) projected
  line L168 (49.854, 34.2607) -> (49.7471, 34.2607) projected
  line L169 (48.3609, 34.1136) -> (48.3609, 31.3369) projected
  line L170 (48.3609, 31.3369) -> (47.0684, 31.3369) projected
  line L171 (47.0684, 35.4864) -> (48.3609, 35.4864) projected
  line L172 (48.3609, 35.4864) -> (48.3609, 34.8891) projected
  line L173 (47.0469, 34.8891) -> (47.0469, 35.2947) projected
  line L174 (50.9728, 37.5277) -> (52.194, 37.5277) projected
  line L175 (52.194, 37.5277) -> (51.0842, 36.0747) projected
  line L176 (51.0842, 36.0747) -> (50.2061, 36.0747) projected
  line L177 (50.2061, 36.0747) -> (50.9728, 37.5277) projected
  line L178 (63.6709, 33.1643) -> (60.8317, 33.1643) projected
  line L179 (60.8317, 33.0592) -> (61.2284, 33.0592) projected
  line L180 (63.4569, 32.6383) -> (63.5951, 32.6383) projected
  line L181 (63.5951, 32.6383) -> (63.5951, 31.5686) projected
  line L182 (64.4108, 32.6472) -> (64.4108, 34.5861) projected
  line L183 (64.4108, 34.5861) -> (63.916, 34.5861) projected
  line L184 (63.916, 34.5861) -> (63.916, 35.4864) projected
  line L185 (63.916, 35.4864) -> (64.4108, 35.4864) projected
  line L186 (64.4108, 35.4864) -> (64.4108, 36.672) projected
  line L187 (64.4108, 36.672) -> (65.7033, 36.672) projected
  line L188 (65.7033, 36.672) -> (65.7033, 35.4864) projected
  line L189 (65.7033, 35.4864) -> (66.9513, 35.4864) projected
  line L190 (66.9513, 35.4864) -> (66.9513, 34.5861) projected
  line L191 (66.9513, 34.5861) -> (65.7033, 34.5861) projected
  line L192 (65.7033, 34.5861) -> (65.7033, 33.1108) projected
  line L193 (66.8398, 32.2818) -> (66.9513, 32.2818) projected
  line L194 (66.9513, 32.2818) -> (66.9513, 31.3725) projected
  line L195 (2.771, 24.9623) -> (1.9485, 24.9623) projected
  line L196 (4.4189, 24.9623) -> (3.5907, 24.9623) projected
  line L197 (3.5907, 24.9623) -> (3.5907, 26.2698) projected
  line L198 (9.8504, 24.9707) -> (10.1823, 24.9707) projected
  line L199 (7.9733, 25.5153) -> (7.9733, 26.301) projected
  line L200 (15.5089, 25.8869) -> (15.5089, 24.9623) projected
  line L201 (15.5089, 24.9623) -> (14.6778, 24.9623) projected
  line L202 (21.9218, 24.7439) -> (22.0182, 24.7439) projected
  line L203 (22.0182, 25.8479) -> (22.3302, 25.8479) projected
  line L204 (17.7829, 24.6418) -> (17.7829, 24.5822) projected
  line L205 (22.7244, 26.2572) -> (23.2832, 26.2572) projected
  line L206 (18.0078, 24.7467) -> (18.0078, 25.2204) projected
  line L207 (23.4108, 25.2204) -> (23.4108, 25.2686) projected
  line L208 (18.5953, 25.2686) -> (18.5953, 24.9991) projected
  line L209 (22.7159, 26.2572) -> (21.6466, 26.2572) projected
  line L210 (19.1626, 26.3492) -> (19.1626, 27.3249) projected
  line L211 (21.97, 25.8479) -> (22.7528, 25.8479) projected
  line L212 (18.5953, 27.6738) -> (18.5953, 27.4866) projected
  line L213 (24.2334, 24.8005) -> (23.8391, 24.8005) projected
  line L214 (19.1626, 24.2447) -> (19.1626, 23.9696) projected
  line L215 (27.9092, 25.5636) -> (27.9801, 25.5636) projected
  line L216 (26.0486, 27.6029) -> (26.3634, 27.6029) projected
  line L217 (27.1859, 27.6029) -> (27.9801, 27.6029) projected
  line L218 (27.9801, 27.6029) -> (27.9801, 27.0299) projected
  line L219 (24.8959, 25.6628) -> (24.8959, 25.4841) projected
  line L220 (27.5859, 24.371) -> (27.9092, 24.371) projected
  line L221 (32.2062, 27.0409) -> (31.3752, 27.0409) projected
  line L222 (35.227, 26.9307) -> (35.227, 26.2755) projected
  line L223 (42.207, 24.8306) -> (42.3517, 24.8306) projected
  line L224 (43.1033, 24.8005) -> (42.7289, 24.8005) projected
  line L225 (33.0969, 27.0952) -> (33.0969, 26.9307) projected
  line L226 (51.147, 28.6183) -> (49.7544, 24.2021) projected
  line L227 (49.7544, 24.2021) -> (49.0794, 24.2021) projected
  line L228 (53.47, 25.7933) -> (53.47, 26.9902) projected
  line L229 (40.9218, 26.9902) -> (40.9218, 27.0555) projected
  line L230 (44.6428, 30.9917) -> (44.654, 31.027) projected
  line L231 (58.876, 23.8281) -> (58.6406, 23.8281) projected
  line L232 (43.9887, 30.4598) -> (44.0972, 30.8045) projected
  line L233 (59.6872, 26.9825) -> (59.3014, 26.9825) projected
  line L234 (63.6211, 27.4421) -> (63.2552, 27.4421) projected
  line L235 (47.6019, 30.0365) -> (47.4269, 29.4725) projected
  line L236 (62.2313, 24.2877) -> (61.1762, 24.2877) projected
  line L237 (45.0378, 26.8569) -> (45.0378, 25.9351) projected
  line L238 (46.0588, 27.0668) -> (46.0588, 27.5546) projected
  line L239 (61.8116, 26.5266) -> (62.1037, 26.5266) projected
  line L240 (69.1803, 28.6183) -> (67.7876, 24.2021) projected
  line L241 (67.7876, 24.2021) -> (67.1126, 24.2021) projected
  line L242 (67.1126, 24.2021) -> (68.5024, 28.6183) projected
  line L243 (68.5024, 28.6183) -> (69.1803, 28.6183) projected
  line L244 (73.1624, 26.908) -> (73.1624, 27.5461) projected
  line L245 (73.1624, 26.9825) -> (74.1069, 26.9825) projected
  line L246 (74.5948, 24.9623) -> (74.5948, 25.2431) projected
  line L247 (52.0381, 25.2431) -> (52.0381, 25.002) projected
  line L248 (76.0214, 24.9623) -> (76.0214, 28.6183) projected
  line L249 (76.0214, 28.6183) -> (76.844, 28.6183) projected
  line L250 (82.5308, 24.9623) -> (82.5308, 27.6029) projected
  line L251 (89.1989, 26.6215) -> (90.1973, 26.6215) projected
  line L252 (68.2365, 33.434) -> (68.3468, 33.7898) projected
  line L253 (67.6087, 27.1576) -> (67.6087, 26.6215) projected
  line L254 (31.6887, 15.882) -> (31.6887, 19.9558) projected
  line L255 (75.3295, 17.3927) -> (75.3295, 15.8251) projected
  line L256 (37.3776, 19.959) -> (38.3478, 19.959) projected
  line L257 (38.3478, 19.959) -> (38.3478, 19.2447) projected
  line L258 (38.3478, 19.2447) -> (37.3776, 19.2447) projected
  line L259 (37.3776, 19.2447) -> (37.3776, 19.959) projected
  line L260 (86.3627, 18.8275) -> (86.3627, 17.8257) projected
  line L261 (46.2332, 24.371) -> (46.584, 24.371) projected
  line L262 (81.3189, 18.9255) -> (81.3189, 19.1278) projected
  line L263 (47.2887, 27.4421) -> (46.565, 27.4421) projected
  line L264 (85.5268, 15.9073) -> (85.5268, 15.8251) projected
  line L265 (56.1696, 24.8306) -> (55.0982, 24.8306) projected
  line L266 (56.8207, 16.552) -> (56.8997, 16.552) projected
  line L267 (56.8997, 16.552) -> (56.8997, 15.9073) projected
  line L268 (86.3068, 17.2599) -> (86.3068, 17.1525) projected
  line L269 (58.2334, 24.8306) -> (57.9774, 24.8306) projected
  line L270 (70.3569, 18.8244) -> (70.3569, 17.9552) projected
  line L271 (70.3569, 17.9552) -> (70.281, 17.9552) projected
  line L272 (69.2981, 17.8509) -> (69.2981, 15.882) projected
  line L273 (69.2981, 15.882) -> (68.3816, 15.882) projected
  line L274 (68.3816, 18.8244) -> (69.2981, 18.8244) projected
  line L275 (69.2981, 18.8244) -> (69.2981, 18.4009) projected
  line L276 (92.1536, 18.4009) -> (92.1536, 18.6885) projected
  line L277 (36.838, 16.4414) -> (36.838, 16.65) projected
  line L278 (73.0306, 15.7473) -> (73.4731, 15.7473) projected
  line L279 (9.7414, 12.6083) -> (9.6024, 12.6083) projected
  line L280 (9.6024, 12.6083) -> (9.6024, 11.4389) projected
  line L281 (40.4093, 10.9048) -> (40.4093, 9.3436) projected
  line L282 (15.7241, 15.7473) -> (14.204, 15.7473) projected
  line L283 (18.7139, 11.7392) -> (18.7139, 9.4352) projected
  line L284 (18.7139, 9.4352) -> (17.7974, 9.4352) projected
  line L285 (19.4124, 12.3776) -> (19.4124, 11.7392) projected
  line L286 (19.4124, 11.7392) -> (18.7139, 11.7392) projected
  line L287 (29.0613, 11.5085) -> (28.9854, 11.5085) projected
  line L288 (48.9985, 11.5085) -> (48.9985, 11.5464) projected
  line L289 (37.4965, 11.6033) -> (37.4175, 11.6033) projected
  line L290 (37.4175, 11.6033) -> (37.4175, 12.3144) projected
  line L291 (61.3096, 12.3144) -> (61.3096, 12.4598) projected
  line L292 (39.0135, 9.4352) -> (39.0135, 9.7481) projected
  line L293 (39.0135, 17.0358) -> (38.6438, 17.0358) projected
  line L294 (43.7068, 9.4352) -> (43.7068, 12.3776) projected
  line L295 (62.9531, 10.9048) -> (62.9531, 9.3436) projected
  line L296 (46.6302, 15.7473) -> (45.11, 15.7473) projected
  line L297 (18.2138, 9.7544) -> (18.2138, 9.4352) projected
  line L298 (51.8165, 9.4352) -> (50.2584, 9.4352) projected
  line L299 (64.0447, 11.5748) -> (64.0447, 10.6299) projected
  line L300 (53.3746, 9.3896) -> (52.9701, 9.3896) projected
  line L301 (65.4444, 13.509) -> (66.3609, 13.509) projected
  line L302 (66.3609, 13.509) -> (66.3609, 9.4352) projected
  line L303 (66.3609, 9.4352) -> (65.4444, 9.4352) projected
  line L304 (65.4444, 9.4352) -> (65.4444, 9.7418) projected
  line L305 (65.4444, 10.8483) -> (65.0399, 10.8483) projected
  line L306 (29.3337, 9.4573) -> (29.3337, 9.353) projected
  line L307 (67.9664, 8.4074) -> (67.0404, 8.4074) projected
  line L308 (39.0509, 9.4415) -> (39.0509, 9.3562) projected
  line L309 (74.831, 8.4074) -> (73.1085, 8.4074) projected
  line L310 (81.4742, 9.4352) -> (80.5324, 9.4352) projected
  line L311 (80.5324, 9.4352) -> (79.028, 12.1532) projected
  line L312 (79.028, 12.1532) -> (79.028, 9.4352) projected
  line L313 (79.028, 9.4352) -> (78.1336, 9.4352) projected
  line L314 (88.9329, 11.5436) -> (90.4499, 11.5436) projected
  line L315 (45.1749, 10.9048) -> (45.1749, 9.3436) projected
  line L316 (88.9329, 10.9941) -> (87.4127, 10.9941) projected
  line L317 (44.4285, 10.9048) -> (44.4285, 12.4693) projected
  line L318 (44.4187, 3.3978) -> (44.4187, 2.6614) projected
  line L319 (44.4187, 2.6614) -> (41.5521, 2.6614) projected
  line L320 (45.091, 4.071) -> (45.091, 3.3978) projected
  line L321 (42.7657, 3.3978) -> (44.4187, 3.3978) projected
  line L322 (54.668, 2.6614) -> (51.8015, 2.6614) projected
  line L323 (52.3419, 9.4042) -> (51.9721, 9.4042) projected
  line L324 (51.9721, 5.5438) -> (51.8963, 5.5438) projected
  line L325 (54.4974, 9.1173) -> (53.7957, 9.1173) projected
  circle A0 centre (94, 20) radius 1.75 projected
  circle A1 centre (6, 20) radius 1.75 projected
  arc A2 (96.5858, 39.4142) -> (95.1716, 40) centre (95.1716, 38) ccw projected
  line L326 (95.1716, 40) -> (4.8284, 40) projected
  arc A3 (4.8284, 40) -> (3.4142, 39.4142) centre (4.8284, 38) ccw projected
  line L327 (0.5858, 36.5858) -> (3.4142, 39.4142) projected
  arc A4 (0.5858, 36.5858) -> (0, 35.1716) centre (2, 35.1716) ccw projected
  line L328 (0, 35.1716) -> (0, 4.8284) projected
  arc A5 (0, 4.8284) -> (0.5858, 3.4142) centre (2, 4.8284) ccw projected
  line L329 (3.4142, 0.5858) -> (0.5858, 3.4142) projected
  arc A6 (3.4142, 0.5858) -> (4.8284, 0) centre (4.8284, 2) ccw projected
  line L330 (4.8284, 0) -> (95.1716, 0) projected
  arc A7 (95.1716, 0) -> (96.5858, 0.5858) centre (95.1716, 2) ccw projected
  line L331 (99.4142, 3.4142) -> (96.5858, 0.5858) projected
  arc A8 (99.4142, 3.4142) -> (100, 4.8284) centre (98, 4.8284) ccw projected
  line L332 (100, 4.8284) -> (100, 35.1716) projected
  arc A9 (100, 35.1716) -> (99.4142, 36.5858) centre (98, 35.1716) ccw projected
  line L333 (96.5858, 39.4142) -> (99.4142, 36.5858) projected
  line L334 (4.8284, 38.6031) -> (95.1716, 38.6031)
  arc A10 (95.5981, 38.4265) -> (95.1716, 38.6031) centre (95.1716, 38) ccw
  line L335 (95.5981, 38.4265) -> (98.4265, 35.5981)
  arc A11 (98.6031, 35.1716) -> (98.4265, 35.5981) centre (98, 35.1716) ccw
  line L336 (98.6031, 35.1716) -> (98.6031, 4.8284)
  arc A12 (98.4265, 4.4019) -> (98.6031, 4.8284) centre (98, 4.8284) ccw
  line L337 (98.4265, 4.4019) -> (95.5981, 1.5735)
  arc A13 (95.1716, 1.3969) -> (95.5981, 1.5735) centre (95.1716, 2) ccw
  line L338 (95.1716, 1.3969) -> (4.8284, 1.3969)
  arc A14 (4.4019, 1.5735) -> (4.8284, 1.3969) centre (4.8284, 2) ccw
  line L339 (4.4019, 1.5735) -> (1.5735, 4.4019)
  arc A15 (1.3969, 4.8284) -> (1.5735, 4.4019) centre (2, 4.8284) ccw
  line L340 (1.3969, 4.8284) -> (1.3969, 35.1716)
  arc A16 (1.5735, 35.5981) -> (1.3969, 35.1716) centre (2, 35.1716) ccw
  line L341 (1.5735, 35.5981) -> (4.4019, 38.4265)
  arc A17 (4.8284, 38.6031) -> (4.4019, 38.4265) centre (4.8284, 38) ccw
  line L342 (51.2721, 6.6404) -> (51.2721, 6.1126) projected
  line L343 (64.9767, 10.0022) -> (65.4444, 10.0022) projected
  line L344 (57.0692, 9.4352) -> (57.0692, 12.3776) projected
  line L345 (52.4592, 24.371) -> (53.4738, 24.371) projected
  line L346 (90.5544, 18.9034) -> (90.5544, 18.6948) projected
  line L347 (52.0895, 16.04) -> (52.0895, 16.8143) projected
  line L348 (52.0895, 16.8143) -> (52.1653, 16.8143) projected
  line L349 (88.8891, 16.8143) -> (88.8891, 16.5773) projected
  line L350 (91.1459, 17.9331) -> (91.1459, 18.6126) projected
  line L351 (72.242, 18.9255) -> (72.242, 19.1309) projected
  line L352 (52.4912, 27.4043) -> (52.4912, 27.6936) projected
  line L353 (50.7266, 25.1948) -> (50.7266, 24.9963) projected
  line L354 (72.1839, 26.2572) -> (71.4833, 26.2572) projected
  line L355 (51.3182, 24.8942) -> (51.3182, 26.7094) projected
  line L356 (72.6689, 28.2382) -> (72.6689, 27.4043) projected
  line L357 (72.6689, 27.4043) -> (72.581, 27.4043) projected
  line L358 (45.6253, 27.2285) -> (45.6253, 27.0668) projected
  line L359 (33.3704, 27.6738) -> (33.3704, 27.2143) projected
  line L360 (46.8387, 25.8479) -> (47.7094, 25.8479) projected
  line L361 (33.1455, 27.6738) -> (33.1455, 27.4384) projected
  line L362 (48.2852, 26.2572) -> (48.5064, 26.2572) projected
  line L363 (48.5064, 26.6811) -> (48.5064, 24.9623) projected
  line L364 (48.5064, 24.9623) -> (47.6782, 24.9623) projected
  line L365 (47.6782, 24.9623) -> (47.6782, 26.2811) projected
  line L366 (47.6782, 26.2572) -> (47.63, 26.2572) projected
  line L367 (34.5252, 26.8286) -> (34.5252, 26.9902) projected
  line L368 (47.3124, 25.8479) -> (46.9295, 25.8479) projected
  line L369 (46.9295, 26.8314) -> (46.9295, 24.9623) projected
  line L370 (67.4772, 31.3369) -> (67.4772, 35.4864) projected
  line L371 (47.0684, 31.3369) -> (47.0684, 35.4864) projected
  line L372 (32.5297, 25.6458) -> (32.5297, 25.47) projected
  line L373 (48.4518, 18.6031) -> (48.3538, 18.6031) projected
  line L374 (48.3538, 25.7) -> (47.9303, 25.7) projected
  line L375 (85.7752, 15.9199) -> (85.7752, 15.8061) projected
  line L376 (47.1307, 26.2572) -> (45.2218, 26.2572) projected
  line L377 (86.3627, 17.8288) -> (86.3627, 19.8578) projected
  line L378 (56.0148, 18.8244) -> (56.8997, 18.8244) projected
  line L379 (56.8997, 18.8244) -> (56.8997, 18.1859) projected
  line L380 (56.4604, 24.9626) -> (56.8207, 24.9626) projected
  line L381 (50.2584, 9.4352) -> (50.2584, 13.3352) projected
  line L382 (50.2584, 13.3352) -> (51.6332, 13.3352) projected
  line L383 (54.3645, 5.8914) -> (54.3645, 5.7618) projected
  line L384 (9.6024, 11.4389) -> (9.6719, 11.4389) projected
  line L385 (51.8015, 2.6614) -> (51.8015, 3.2967) projected
  line L386 (41.5521, 2.6614) -> (41.5521, 3.2967) projected
  line L387 (41.7228, 5.5438) -> (41.6469, 5.5438) projected
  line L388 (81.4742, 13.3352) -> (81.4742, 9.4352) projected
  line L389 (78.1336, 9.4352) -> (78.1336, 13.3352) projected
  line L390 (78.1336, 13.3352) -> (79.3346, 13.3352) projected
  line L391 (79.3346, 13.3352) -> (80.5798, 11.1008) projected
  line L392 (80.5798, 11.1008) -> (80.5798, 13.3352) projected
  line L393 (80.5798, 13.3352) -> (81.4742, 13.3352) projected
  line L394 (76.0382, 11.0629) -> (76.0382, 10.731) projected
  line L395 (76.0382, 10.731) -> (74.025, 10.731) projected
  line L396 (75.8865, 10.3581) -> (75.9845, 10.3581) projected
  line L397 (69.7932, 12.3776) -> (69.7932, 9.4352) projected
  line L398 (67.0404, 10.4624) -> (67.0404, 12.3776) projected
  line L399 (67.0404, 12.3776) -> (67.9633, 12.3776) projected
  line L400 (67.9633, 12.3776) -> (67.9633, 10.9175) projected
  line L401 (68.8767, 10.2917) -> (68.8767, 12.3776) projected
  line L402 (68.8767, 12.3776) -> (69.7932, 12.3776) projected
  line L403 (63.2163, 11.0629) -> (63.2163, 10.731) projected
  line L404 (63.2163, 10.731) -> (61.2031, 10.731) projected
  line L405 (63.0646, 10.3581) -> (63.1626, 10.3581) projected
  line L406 (39.0199, 11.3663) -> (39.0199, 11.3821) projected
  line L407 (19.6083, 13.4806) -> (19.6083, 12.8169) projected
  line L408 (19.6083, 12.8169) -> (19.5388, 12.8169) projected
  line L409 (18.6823, 12.3997) -> (18.6823, 12.3776) projected
  line L410 (18.6823, 12.3776) -> (19.4124, 12.3776) projected
  line L411 (17.7974, 9.4352) -> (17.7974, 11.7392) projected
  line L412 (17.7974, 11.7392) -> (17.4308, 11.7392) projected
  line L413 (17.4308, 11.7392) -> (17.4308, 12.3776) projected
  line L414 (17.4308, 12.3776) -> (17.7974, 12.3776) projected
  line L415 (17.7974, 12.3776) -> (17.7974, 12.4598) projected
  line L416 (55.0982, 16.8111) -> (55.0982, 18.1859) projected
  line L417 (55.0982, 18.1859) -> (54.7474, 18.1859) projected
  line L418 (54.7474, 18.1859) -> (54.7474, 18.8244) projected
  line L419 (54.7474, 18.8244) -> (55.0982, 18.8244) projected
  line L420 (55.0982, 18.8244) -> (55.0982, 19.665) projected
  line L421 (48.3633, 17.0577) -> (48.4518, 17.0577) projected
  line L422 (48.4518, 17.0577) -> (48.4518, 16.1411) projected
  line L423 (74.6004, 26.6952) -> (74.6004, 26.7094) projected
  line L424 (73.2333, 26.908) -> (73.1624, 26.908) projected
  line L425 (61.4967, 26.7406) -> (61.4967, 26.7548) projected
  line L426 (31.3752, 25.8841) -> (31.3752, 27.6029) projected
  line L427 (31.3752, 27.6029) -> (32.2034, 27.6029) projected
  line L428 (32.2034, 27.6029) -> (32.2034, 26.2925) projected
  line L429 (33.0231, 25.7309) -> (33.0231, 27.6029) projected
  line L430 (33.0231, 27.6029) -> (33.8456, 27.6029) projected
  line L431 (26.3634, 25.7961) -> (26.3634, 27.0299) projected
  line L432 (26.3634, 27.0299) -> (26.0486, 27.0299) projected
  line L433 (26.0486, 27.0299) -> (26.0486, 27.6029) projected
  line L434 (7.0765, 25.7961) -> (7.0765, 27.0299) projected
  line L435 (7.0765, 27.0299) -> (6.7617, 27.0299) projected
  line L436 (6.7617, 27.0299) -> (6.7617, 27.6029) projected
  line L437 (6.7617, 27.6029) -> (7.0765, 27.6029) projected
  line L438 (7.0765, 27.6029) -> (7.0765, 28.3573) projected
  line L439 (7.0765, 28.3573) -> (7.8991, 28.3573) projected
  line L440 (7.8991, 28.3573) -> (7.8991, 27.6029) projected
  line L441 (7.8991, 27.6029) -> (8.6932, 27.6029) projected
  line L442 (8.6932, 27.6029) -> (8.6932, 27.0299) projected
  line L443 (8.6932, 27.0299) -> (7.8991, 27.0299) projected
  line L444 (7.8991, 27.0299) -> (7.8991, 26.0911) projected
  line L445 (4.4189, 26.6811) -> (4.4189, 24.9623) projected
  line L446 (1.9485, 24.9623) -> (1.9485, 28.6183) projected
  line L447 (1.9485, 28.6183) -> (2.771, 28.6183) projected
  line L448 (2.771, 28.6183) -> (2.771, 27.3107) projected
  line L449 (11.8812, 25.1041) -> (11.8812, 25.799) projected
  line L450 (11.8812, 25.799) -> (11.9493, 25.799) projected
  line L451 (34.4752, 24.9623) -> (34.4752, 28.6183) projected
  line L452 (34.4752, 28.6183) -> (35.2978, 28.6183) projected
  line L453 (35.2978, 28.6183) -> (35.2978, 27.3249) projected
  line L454 (44.5243, 24.9623) -> (44.5243, 27.6029) projected
  line L455 (44.5243, 27.6029) -> (45.3468, 27.6029) projected
  line L456 (45.3468, 27.6029) -> (45.3468, 27.3107) projected